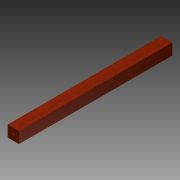
# Autodesk Inventor part: WoodColumn
Saved by Autodesk Inventor 2014 SP1 (Build 180222100, 222)
## iProperties
Created: 2015-05-01
Part Number: WoodColumn
Material: Wood (Oak)
Document SubType Name: Modeling
Designer: david
Mass: 76.874 g
Surface Area: 243.78 cm^2
Volume: 101.15 cm^3
Density: 0.76 g/cm^3
Appearance: White Oak - Natural Medium Gloss
Author: david
Autodesk Inventor part; units mm, degrees
ref_plane "YZ Plane" through (0, 0, 0) normal (1, 0, 0) x (0, 1, 0)
ref_plane "XZ Plane" through (0, 0, 0) normal (0, 1, 0) x (-1, 0, 0)
ref_plane "XY Plane" through (0, 0, 0) normal (0, 0, 1) x (1, 0, 0)
sketch "Sketch1" plane through (0, 0, 0) normal (0, 1, 0) x (-1, 0, 0)
  line L0 (-8.5, 8.5) -> (8.5, 8.5)
  line L1 (8.5, 8.5) -> (8.5, -8.5)
  line L2 (8.5, -8.5) -> (-8.5, -8.5)
  line L3 (-8.5, -8.5) -> (-8.5, 8.5)
  line L4 (-8.5, 8.5) -> (8.5, -8.5) construction
  line L5 (8.5, 8.5) -> (-8.5, -8.5) construction
  point P0 (0, 0)
  dimension "d0" = 17
  dimension "d1" = 17
  constraints: 12 end point, 2 midpoint, 2 parallel, 1 horizontal, 1 perpendicular
  measures "d0" distance of L1.end L2.end
  measures "d1" distance of L0.end L1.end
extrude "Extrusion1" add sketch "Sketch1" along normal blind 230
sketch "Sketch2" plane through (0, 0, 0) normal (0, -1, 0) x (1, 0, 0)
  circle A0 centre (0, 0) radius 1.5
  dimension "d4" = 3
  constraints: 1 centre point, 1 coincident
  measures "d4" diameter of A0
extrude "Extrusion2" cut sketch "Sketch2" against normal blind 20
body "Solid1"
